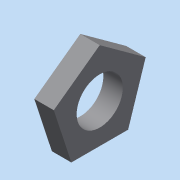
# Autodesk Inventor part: Bracket
Saved by Autodesk Inventor 2015 (Build 190159000, 159)
## iProperties
Created: 2014-09-21
Part Number: Bracket
Material: Generic
Document SubType Name: Modeling
Designer: Kris
Density: 1 g/cm^3
Appearance: Default
Author: Kris
Autodesk Inventor part; units mm, degrees
ref_plane "YZ Plane" through (0, 0, 0) normal (1, 0, 0) x (0, 1, 0)
ref_plane "XZ Plane" through (0, 0, 0) normal (0, 1, 0) x (-1, 0, 0)
ref_plane "XY Plane" through (0, 0, 0) normal (0, 0, 1) x (1, 0, 0)
sketch "Sketch1" plane through (0, 0, 0) normal (1, 0, 0) x (0, 1, 0)
  circle A0 centre (0, 0) radius 2.5
  line L0 (5.2285, 0) -> (1.6157, -4.9726)
  line L1 (1.6157, -4.9726) -> (-4.23, -3.0733)
  line L2 (-4.23, -3.0733) -> (-4.23, 3.0733)
  line L3 (-4.23, 3.0733) -> (1.6157, 4.9726)
  line L4 (1.6157, 4.9726) -> (5.2285, 0)
  dimension "d0" = 5
  constraints: 10 end point, 2 coincident, 1 centre point, 11 other
  measures "d0" diameter of A0
extrude "Extrusion1" add sketch "Sketch1" along normal blind 2.1082
body "Solid1"
